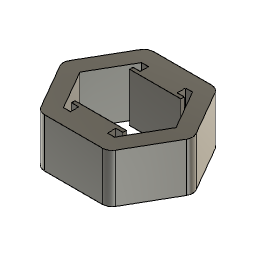
Hotwheels-makeshift-tunnel-adapter v2 (Autodesk Fusion 360 design; units mm, degrees)
Autodesk Fusion 360 part; units mm, degrees
sketch "Sketch1" plane through (0, 0, 0) normal (0, 0, 1) x (1, 0, 0)
  line L0 (0, 0) -> (0, 40)
  line L1 (0, 40) -> (-13.1, 40)
  line L2 (0, 40) -> (13.1, 40)
  line L3 (0, 0) -> (-13.1, 0)
  line L4 (0, 0) -> (13.1, 0)
  line L5 (0, 20) -> (24.647, 20)
  line L6 (0, 20) -> (-24.647, 20)
  line L7 (13.1, 40) -> (24.647, 20)
  line L8 (-13.1, 40) -> (-24.647, 20)
  line L9 (-13.1, 0) -> (-24.647, 20)
  line L10 (13.1, 0) -> (24.647, 20)
  line L11 (0, 40) -> (0, 34)
  line L12 (0, 0) -> (0, 6)
  line L13 (0, 6) -> (13.15, 6)
  line L14 (0, 6) -> (-13.15, 6)
  line L15 (0, 34) -> (13.15, 34)
  line L16 (0, 34) -> (-13.15, 34)
  line L17 (-13.15, 34) -> (-13.15, 35.75)
  line L18 (13.15, 34) -> (13.15, 35.75)
  line L19 (-13.15, 6) -> (-13.15, 4.25)
  line L20 (13.15, 6) -> (13.15, 4.25)
  line L21 (-13.15, 4.25) -> (13.15, 4.25)
  line L22 (-13.15, 35.75) -> (13.15, 35.75)
  line L23 (0, 35.75) -> (-9.5, 35.75)
  line L24 (0, 35.75) -> (9.5, 35.75)
  line L25 (9.5, 35.75) -> (9.5, 40)
  line L26 (-9.5, 35.75) -> (-9.5, 40)
  line L27 (-9.5, 40) -> (-9.5, 0)
  line L28 (9.5, 40) -> (9.5, 0)
  line L29 (0, 48) -> (-17.7188, 48)
  line L30 (-17.7188, 48) -> (-33.8846, 20)
  line L31 (-17.7188, -8) -> (-33.8846, 20)
  line L32 (0, -8) -> (-17.7188, -8)
  line L33 (0, -8) -> (17.7188, -8)
  line L34 (17.7188, -8) -> (33.8846, 20)
  line L35 (17.7188, 48) -> (33.8846, 20)
  line L36 (0, 48) -> (17.7188, 48)
  dimension "d1" = 40
  dimension "d2" = 13.1
  dimension "d3" = 13.1
  dimension "d4" = 13.1
  dimension "d5" = 13.1
  dimension "d11" = 6
  dimension "d12" = 6
  dimension "d13" = 13.15
  dimension "d14" = 13.15
  dimension "d15" = 13.15
  dimension "d16" = 13.15
  dimension "d17" = 1.75
  dimension "d18" = 1.75
  dimension "d19" = 1.75
  dimension "d20" = 1.75
  dimension "d21" = 9.5
  dimension "d22" = 9.5
  dimension "d23" = 8
  constraint coincident L0.start L3.start
  constraint vertical L0
  constraint perpendicular L0 L1
  constraint perpendicular L0 L2
  constraint perpendicular L0 L3
  constraint perpendicular L0 L4
  constraint midpoint L0 L5.start
  constraint perpendicular L0 L5
  constraint perpendicular L0 L6
  constraint perpendicular L4 L12
  constraint perpendicular L0 L13
  constraint perpendicular L12 L14
  constraint perpendicular L11 L15
  constraint perpendicular L11 L16
  constraint perpendicular L16 L17
  constraint perpendicular L15 L18
  constraint perpendicular L14 L19
  constraint perpendicular L13 L20
  constraint midpoint L22 L23.start
  constraint perpendicular L11 L23
  constraint perpendicular L0 L24
  constraint coincident L2 L25.end
  constraint coincident L3 L27.end
  constraint perpendicular L3 L27
  constraint coincident L4 L28.end
  constraint perpendicular L4 L28
  measures "d1" distance of L0.start L0.end
  measures "d2" distance of L0.end L1.end
  measures "d3" distance of L0.end L2.end
  measures "d4" distance of L0.start L3.end
  measures "d5" distance of L0.start L4.end
  measures "d11" distance of L0.end L11.end
  measures "d12" distance of L0.start L12.end
  measures "d13" distance of L12.end L13.end
  measures "d14" distance of L12.end L14.end
  measures "d15" distance of L11.end L15.end
  measures "d16" distance of L11.end L16.end
  measures "d17" distance of L16.end L17.end
  measures "d18" distance of L15.end L18.end
  measures "d19" distance of L14.end L19.end
  measures "d20" distance of L13.end L20.end
  measures "d21" distance of L23.start L23.end
  measures "d22" distance of L23.start L24.end
extrude "Extrude1" add sketch "Sketch1" along normal blind 25 contours L0 L12 L13 L21 L28 | L0 L12 L14 L21 L27 | L0 L4 L12 L21 L28 | L0 L3 L12 L21 L27 | L13 L20 L21 L28 | L14 L19 L21 L27 | L0 L11 L16 L22 L23 L27 | L0 L11 L15 L22 L24 L28 | L0 L1 L11 L22 L23 L26 L27 | L0 L2 L11 L22 L24 L25 L28 | L15 L18 L22 L28 | L16 L17 L22 L27 | L29 L30 L31 L32 L33 L34 L35 L36
fillet "Fillet1" radius 5 6 edges at (-33.8846, 20, 12.5) (-17.7188, -8, 12.5) (17.7188, -8, 12.5) (-17.7188, 48, 12.5) (17.7188, 48, 12.5) (33.8846, 20, 12.5)
equation "d21 = ( 19 / 2 ) * 1 mm"
equation "d22 = ( 19 / 2 ) * 1 mm"
